Tube OLD (Autodesk Fusion 360 design; units mm, degrees)
Autodesk Fusion 360 part; units mm, degrees
ref_plane "WorkPlane1" through (0, 60, 0) normal (0, 1, 0) x (0, 0, 1)
sketch "Sketch1" plane through (0, 60, 0) normal (0, 1, 0) x (1, 0, 0)
  line L0 (20, 28.7228) -> (20, -28.7228)
  line L1 (25, 24.4949) -> (25, -24.4949)
  arc A0 (25, 24.4949) -> (25, -24.4949) centre (0, 0) ccw
  arc A1 (25, 16.5831) -> (25, -16.5831) centre (0, 0) ccw
  dimension "d2" = 60
  dimension "d3" = 70
  dimension "d4" = 20
  dimension "d5" = 5
  constraint coincident A0.centre A1.centre
  constraint concentric A0 A1
  constraint coincident L0.start A0
  constraint coincident L0.end A0
  constraint vertical L0
  constraint vertical L1
  constraint coincident L1 A1.end
  constraint coincident L1 A1.start
  measures "d2" diameter of A1
  measures "d3" diameter of A0
  measures "d4" distance of A0.centre L0
  measures "d5" distance of L0 L1
extrude "Extrude1" add sketch "Sketch1" along normal blind 100 contours L0 L1 A0 A1 | L0 A0 A1 | L0 L1 A1 | L0 L1 A0 A1
extrude "Extrude2" add sketch "Sketch1" against normal blind 60 contours L0 L1 A0 A1 | L0 L1 A1 | L0 L1 A0 A1
ref_plane "WorkPlane2" through (0, 124.607, 35) normal (0, 0, 1) x (-1, 0, 0)
sketch "Sketch2" plane through (0, 124.607, 35) normal (0, 0, 1) x (1, 0, 0)
  line L0 (20, -64.607) -> (-35, -64.607)
  line L1 (20, -64.607) -> (20, -124.607)
  line L2 (20, -124.607) -> (25, -124.607)
  line L3 (25, -124.607) -> (25, 35.393)
  line L4 (25, 35.393) -> (-35, 35.393)
  line L5 (25, 35.393) -> (25, -124.607)
  line L6 (20, -124.607) -> (25, -124.607)
  line L7 (20, -124.607) -> (20, -64.607)
  line L8 (-10, -9.607) -> (10, -9.607)
  line L9 (10, -9.607) -> (10, -19.607)
  line L10 (10, -19.607) -> (-10, -19.607)
  line L11 (-10, -19.607) -> (-10, -9.607)
  dimension "d11" = 45
  dimension "d12" = 10
  dimension "d13" = 20
  dimension "d14" = 15
  constraint horizontal L8
  constraint vertical L9
  constraint horizontal L10
  constraint vertical L11
  measures "d11" distance of L4 L8
  measures "d12" distance of L8.end L9.end
  measures "d13" distance of L9 L11
  measures "d14" distance of L5 L9
ref_plane "WorkPlane3" through (0, 127.6389, 35) normal (0, 0, 1) x (-1, 0, 0)
sketch "Sketch6" plane through (0, 127.6389, 35) normal (0, 0, 1) x (1, 0, 0)
  line L0 (20, -127.6389) -> (25, -127.6389)
  line L1 (20, -67.6389) -> (20, -127.6389)
  line L2 (25, 32.3611) -> (25, -127.6389)
  line L3 (20, -67.6389) -> (-35, -67.6389)
  line L4 (25, 32.3611) -> (-35, 32.3611)
  line L5 (-35, -67.6389) -> (-35, 32.3611)
  line L6 (25, 32.3611) -> (20, 32.3611)
  line L7 (20, 32.3611) -> (20, -127.6389)
  line L8 (20, -127.6389) -> (25, -127.6389)
  line L9 (25, -127.6389) -> (25, 32.3611)
  constraint horizontal L6
  constraint vertical L7
  constraint horizontal L8
  constraint vertical L9
  constraint coincident L0.start L1.end
  constraint coincident L2.start L4.start
extrude "Extrude9" add sketch "Sketch6" against normal blind 15 contours L0 L1 L2 L4 L6 L7 L8 L9
extrude "Extrude10" add sketch "Sketch6" along normal blind 5 contours L0 L1 L2 L4 L6 L7 L8 L9
mirror "Mirror2" about plane through (0, 0, 0) normal (0, 0, 1) of bodies 1 merged
sketch "Sketch7" plane through (25, 0, 0) normal (1, 0, 0) x (0, 0, -1)
  line L0 (40, 160) -> (-40, 160)
  line L1 (-40, 160) -> (-40, 0)
  line L2 (-40, 0) -> (40, 0)
  line L3 (40, 0) -> (40, 160)
  line L4 (-30, 40) -> (30, 40)
  line L5 (30, 40) -> (30, 30)
  line L6 (30, 30) -> (-30, 30)
  line L7 (-30, 30) -> (-30, 40)
  line L8 (28.7228, 160) -> (28.7228, 60)
  line L9 (35, 60) -> (-35, 60)
  line L10 (-28.7228, 60) -> (-28.7228, 160)
  line L11 (35, 160) -> (-35, 160)
  dimension "d41" = 60
  dimension "d42" = 10
  dimension "d43" = 10
  dimension "d45" = 20
  constraint horizontal L4
  constraint vertical L5
  constraint horizontal L6
  constraint vertical L7
  measures "d41" distance of L4.start L4.end
  measures "d42" distance of L3 L5
  measures "d43" distance of L4 L6
  measures "d45" distance of L4 L9
extrude "Extrude11" cut sketch "Sketch7" against normal through all contours L4 L5 L6 L7
sketch "Sketch8" plane through (20, 0, 0) normal (-1, 0, 0) x (0, 0, 1)
  line L0 (30, 40) -> (30, 30)
  line L1 (30, 30) -> (-30, 30)
  line L2 (-30, 30) -> (-30, 40)
  line L3 (-30, 40) -> (30, 40)
  line L4 (-40, 0) -> (40, 0)
  line L5 (40, 0) -> (40, 160)
  line L6 (40, 160) -> (28.7228, 160)
  line L7 (28.7228, 160) -> (28.7228, 60)
  line L8 (28.7228, 60) -> (22.3607, 60)
  line L9 (22.3607, 60) -> (22.3607, 160)
  line L10 (22.3607, 160) -> (-22.3607, 160)
  line L11 (-22.3607, 160) -> (-22.3607, 60)
  line L12 (-22.3607, 60) -> (-28.7228, 60)
  line L13 (-28.7228, 60) -> (-28.7228, 160)
  line L14 (-28.7228, 160) -> (-40, 160)
  line L15 (-40, 160) -> (-40, 0)
  line L16 (-40, 5) -> (40, 5)
  line L17 (40, 5) -> (40, 0)
  line L18 (40, 0) -> (-40, 0)
  line L19 (-40, 0) -> (-40, 5)
  dimension "d47" = 5
  constraint horizontal L16
  constraint vertical L17
  constraint horizontal L18
  constraint vertical L19
  constraint coincident L4.end L5.start
  constraint coincident L15 L16.start
  measures "d47" distance of L16 L18
extrude "Extrude12" add sketch "Sketch8" along normal blind 55 contours L4 L5 L15 L16 L17 L18 L19
sketch "Sketch9" plane through (0, 5, 0) normal (0, 1, 0) x (-1, 0, 0)
  line L0 (-20, 40) -> (-20, -40)
  line L1 (-20, -40) -> (35, -40)
  line L2 (35, -40) -> (35, 40)
  line L3 (35, 40) -> (-20, 40)
  circle A0 centre (-15, 35) radius 3.225
  circle A1 centre (30, 35) radius 3.225
  circle A2 centre (30, -35) radius 3.225
  circle A3 centre (-15, -35) radius 3.225
  dimension "d50" = 6.45
  dimension "d51" = 5
  dimension "d52" = 5
  dimension "d53" = 6.45
  dimension "d54" = 5
  dimension "d57" = 6.45
  dimension "d58" = 6.45
  dimension "d59" = 5
  dimension "d60" = 5
  dimension "d61" = 5
  dimension "d62" = 5
  constraint horizontal A0.centre A1.centre
  measures "d50" diameter of A0
  measures "d51" distance of L3 A0.centre
  measures "d52" distance of L0 A0.centre
  measures "d53" diameter of A1
  measures "d54" distance of L2 A1.centre
  measures "d57" diameter of A3
  measures "d58" diameter of A2
  measures "d59" distance of L2 A2.centre
  measures "d60" distance of L1 A2.centre
  measures "d61" distance of L0 A3.centre
  measures "d62" distance of L1 A3.centre
extrude "Extrude13" cut sketch "Sketch9" against normal blind 5 contours A0 | A1 | A2 | A3
